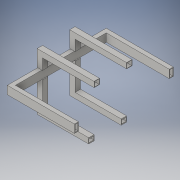
# Autodesk Inventor part: ShooterFrameV03
Saved by Autodesk Inventor 2016 SP1 (Build 200210100, 210)
## iProperties
Created: 2016-01-24
Part Number: ShooterFrameV03
Material: Generic
Document SubType Name: Modeling
Designer: steele
Density: 1 g/cm^3
Appearance: Default
Author: steele
Autodesk Inventor part; units mm, degrees
ref_plane "XZ Plane" through (0, 0, 0) normal (0, 1, 0) x (-1, 0, 0)
sketch "Sketch10" plane through (0, 0, 0) normal (0, 1, 0) x (-1, 0, 0)
  line L0 (0, 0) -> (0, 222.25)
  line L1 (0, 222.25) -> (-304.8, 222.25)
  line L2 (0, 0) -> (-304.8, 0) construction
  line L3 (0, 0) -> (0, -222.25)
  line L4 (0, -222.25) -> (-304.8, -222.25)
  dimension "d31" = 222.25
  dimension "d32" = 304.8
  constraints: 10 end point, 2 symmetric about line, 1 horizontal, 1 perpendicular, 1 vertical
  measures "d31" distance of L0.start L0.end
  measures "d32" distance of L0.end L1.end
ref_plane "Work Plane2" through (304.8, 0, 0) normal (1, 0, 0) x (0, 1, 0)
sketch "Sketch11" plane through (304.8, 0, 0) normal (1, 0, 0) x (0, 1, 0)
  line L0 (-19.05, 231.775) -> (-19.05, 212.725)
  line L1 (-19.05, 212.725) -> (19.05, 212.725)
  line L2 (19.05, 212.725) -> (19.05, 231.775)
  line L3 (19.05, 231.775) -> (-19.05, 231.775)
  line L4 (-19.05, 231.775) -> (19.05, 212.725) construction
  line L5 (-19.05, 212.725) -> (19.05, 231.775) construction
  line L6 (-15.875, 228.6) -> (-15.875, 215.9)
  line L7 (-15.875, 215.9) -> (15.875, 215.9)
  line L8 (15.875, 215.9) -> (15.875, 228.6)
  line L9 (15.875, 228.6) -> (-15.875, 228.6)
  line L10 (-15.875, 228.6) -> (15.875, 215.9) construction
  line L11 (-15.875, 215.9) -> (15.875, 228.6) construction
  point P0 (0, 0)
  point P1 (0, 222.25)
  dimension "d34" = 222.25
  dimension "d35" = 19.05
  dimension "d36" = 38.1
  dimension "d37" = 3.175
  dimension "d38" = 3.175
  constraints: 24 end point, 4 midpoint, 4 parallel, 2 perpendicular, 2 vertical
  measures "d34" distance of point (0, 0) point (0, 222.25)
  measures "d35" distance of L1.end L2.end
  measures "d36" distance of L2.end L0.start
  measures "d37" distance between parallel lines of L3 L9
  measures "d38" distance between parallel lines of L0 L6
sweep "Sweep5" add profiles "Sketch11" path "Sketch10" path curves L1 L0 L3 L4
sketch "Sketch12" plane through (304.8, 19.05, 231.775) normal (0, 1, 0) x (1, 0, 0)
  line L0 (-304.8, 231.775) -> (-304.8, 0) construction
  line L1 (0, 0) -> (-314.325, 0) construction
  line L2 (-317.5, 142.875) -> (-292.1, 142.875)
  line L3 (-292.1, 142.875) -> (-292.1, 168.275)
  line L4 (-292.1, 168.275) -> (-317.5, 168.275)
  line L5 (-317.5, 168.275) -> (-317.5, 142.875)
  line L6 (-317.5, 142.875) -> (-292.1, 168.275) construction
  line L7 (-292.1, 142.875) -> (-317.5, 168.275) construction
  line L8 (-298.45, 15.875) -> (-298.45, 447.675) projected
  line L9 (-315.9125, 144.4625) -> (-293.6875, 144.4625)
  line L10 (-293.6875, 144.4625) -> (-293.6875, 166.6875)
  line L11 (-293.6875, 166.6875) -> (-315.9125, 166.6875)
  line L12 (-315.9125, 166.6875) -> (-315.9125, 144.4625)
  line L13 (-315.9125, 144.4625) -> (-293.6875, 166.6875) construction
  line L14 (-293.6875, 144.4625) -> (-315.9125, 166.6875) construction
  point P0 (-304.8, 155.575)
  dimension "d41" = 25.4
  dimension "d42" = 25.4
  dimension "d43" = 76.2
  dimension "d44" = 1.5875
  dimension "d45" = 1.5875
  constraints: 26 end point, 4 midpoint, 4 parallel, 4 perpendicular, 2 point on line, 1 vertical
  measures "d41" distance of L4.end L2.start
  measures "d42" distance of L2.start L2.end
  measures "d43" distance of point (-304.8, 155.575) L0.start
  measures "d44" distance between parallel lines of L5 L12
  measures "d45" distance between parallel lines of L2 L9
ref_plane "Work Plane3" through (0, 0, 63.5) normal (0, 0, 1) x (1, 0, 0)
sketch "Sketch13" plane through (0, 0, 63.5) normal (0, 0, 1) x (1, 0, 0)
  line L0 (304.8, 19.05) -> (-9.525, 19.05) projected
  line L1 (0, 19.05) -> (0, 82.55)
  line L2 (0, 82.55) -> (254, 82.55)
  point P0 (0, 0)
  dimension "d47" = 254
  dimension "d48" = 63.5
  constraints: 4 end point, 1 perpendicular, 1 point on line, 1 vertical
  measures "d47" distance of L1.end L2.end
  measures "d48" distance of L1.start L1.end
sweep "Sweep6" add profiles "Sketch12" path "Sketch13" path curves L1 L2 contours L5 L4 L8 L11 L12 L9 L2 | L8 L9 L10 L11 L4 L3 L2
mirror "Mirror2" about plane through (0, 0, 0) normal (0, 0, 1) of "Sweep6"
sketch "Sketch14" plane through (304.8, -19.05, 212.725) normal (0, -1, 0) x (1, 0, 0)
  line L0 (-304.8, -212.725) -> (-304.8, 15.875) construction
  line L1 (0, 15.875) -> (-311.15, 15.875) construction
  line L2 (-317.5, -123.825) -> (-317.5, -149.225)
  line L3 (-317.5, -149.225) -> (-292.1, -149.225)
  line L4 (-292.1, -149.225) -> (-292.1, -123.825)
  line L5 (-292.1, -123.825) -> (-317.5, -123.825)
  line L6 (-317.5, -123.825) -> (-292.1, -149.225) construction
  line L7 (-317.5, -149.225) -> (-292.1, -123.825) construction
  line L8 (-312.7375, -125.4125) -> (-312.7375, -147.6375)
  line L9 (-312.7375, -147.6375) -> (-296.8625, -147.6375)
  line L10 (-296.8625, -147.6375) -> (-296.8625, -125.4125)
  line L11 (-296.8625, -125.4125) -> (-312.7375, -125.4125)
  line L12 (-312.7375, -125.4125) -> (-296.8625, -147.6375) construction
  line L13 (-312.7375, -147.6375) -> (-296.8625, -125.4125) construction
  line L14 (-314.325, 19.05) -> (-314.325, -444.5) projected
  point P0 (-304.8, -136.525)
  dimension "d52" = 76.2
  dimension "d53" = 25.4
  dimension "d54" = 25.4
  dimension "d55" = 1.5875
  dimension "d56" = 1.5875
  constraints: 26 end point, 5 parallel, 4 midpoint, 2 perpendicular, 2 point on line, 1 vertical
  measures "d52" distance of point (-304.8, -136.525) L0.start
  measures "d53" distance of L4.end L2.start
  measures "d54" distance of L2.start L2.end
  measures "d55" distance between parallel lines of L5 L11
  measures "d56" distance between parallel lines of L8 L14
ref_plane "Work Plane5" through (0, 0, 76.2) normal (0, 0, 1) x (1, 0, 0)
sketch "Sketch15" plane through (0, 0, 76.2) normal (0, 0, 1) x (1, 0, 0)
  line L0 (-9.525, -19.05) -> (304.8, -19.05) projected
  line L1 (0, -19.05) -> (0, -158.75)
  line L2 (0, -158.75) -> (228.6, -158.75)
  point P0 (0, 0)
  dimension "d58" = 228.6
  dimension "d59" = 139.7
  constraints: 4 end point, 1 perpendicular, 1 point on line, 1 vertical
  measures "d58" distance of L1.end L2.end
  measures "d59" distance of L1.start L1.end
sweep "Sweep7" add profiles "Sketch14" path "Sketch15" path curves L1 L2
mirror "Mirror5" about plane through (0, 0, 0) normal (0, 0, 1) of "Sweep7"
ref_plane "Work Plane6" through (152.4, 0, 0) normal (1, 0, 0) x (0, 1, 0)
equation "\"d31\" = halfOfWidth"
equation "\"d32\" = length"
equation "\"d34\" = halfOfWidth"
equation "\"d35\" = largeTubingWidth"
equation "\"d36\" = largeTubingHeight"
equation "\"d37\" = largeTubeThickness"
equation "\"d38\" = largeTubeThickness"
equation "\"d41\" = smallSupportTubeWidth"
equation "\"d42\" = smallSupportTubeWidth"
equation "\"d43\" = distaceToMiddleSmallSupportTube"
equation "\"d44\" = smallSupportTubeThickness"
equation "\"d45\" = smallSupportTubeThickness"
equation "\"d47\" = topSupportTubeExtension"
equation "\"d48\" = smallSupportTubeLength"
equation "\"d52\" = distaceToMiddleSmallSupportTube"
equation "\"d53\" = smallSupportTubeWidth"
equation "\"d54\" = smallSupportTubeHeight"
equation "\"d55\" = smallSupportTubeThickness"
equation "\"d56\" = smallSupportTubeThickness"
equation "\"d58\" = bottomSupportTubeExtension"
equation "\"halfOfWidth\" = 0.5 * width"
equation "\"length\" = 304.8"
equation "\"height\" = 241.3"
equation "\"largeTubingWidth\" = 19.05"
equation "\"largeTubingHeight\" = 38.1"
equation "\"largeTubeThickness\" = 3.175"
equation "\"d33\" = length"
equation "\"width\" = 444.5"
equation "\"smallSupportTubeWidth\" = 25.4"
equation "\"smallSupportTubeHeight\" = 25.4"
equation "\"smallSupportTubeThickness\" = 1.5875"
equation "\"distaceToMiddleSmallSupportTube\" = 76.2"
equation "\"smallSupportTubeLength\" = 63.5"
equation "\"d46\" = smallSupportTubeLength"
equation "\"d57\" = distaceToMiddleSmallSupportTube"
equation "\"distanceOriginToPlaneForSupportTubes\" = 152.4"
equation "\"d62\" = distanceOriginToPlaneForSupportTubes"
equation "\"topSupportTubeExtension\" = 254"
equation "\"bottomSupportTubeExtension\" = 228.6"
body "Solid5"
